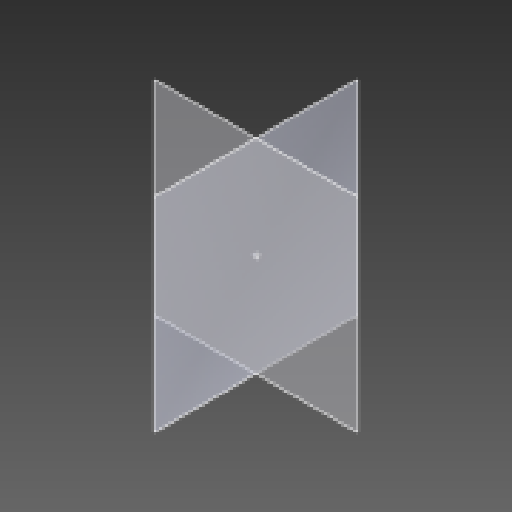
# Autodesk Inventor part: DrumstickBoundingBox
Saved by Autodesk Inventor 2023 (Build 270158000, 158)
## iProperties
Created: 2023-03-24
Part Number: DrumstickBoundingBox
Material: Generic
Document SubType Name: Modeling
Designer: Val
Density: 1 g/cm^3
Appearance: Default
Author: Val
Autodesk Inventor part; units mm, degrees
sketch "Base" plane through (0, 0, 0) normal (0, 1, 0) x (-1, 0, 0)
  arc A0 (16.4327, -16.6683) -> (16.4327, -3.9692) centre (16.3612, -10.3188) ccw projected
  circle A1 centre (16.3612, -10.3188) radius 6.35
  point P0 (0, 0)
  constraints: 1 coincident, 3 other
extrude "ForwardFeature" add sketch "Base" along normal blind 309.88 draft -0.5
sketch "Sketch2" plane through (-16.3612, 0, -10.3188) normal (0, -1, 0) x (1, 0, 0)
  circle A0 centre (0, 0) radius 6.35 projected
  point P0 (16.3612, 10.3188)
extrude "BackFeature" add sketch "Sketch2" along normal blind 88.9
sketch "Sketch3" plane through (0, 0, 0) normal (0, 1, 0) x (-1, 0, 0)
  arc A0 (16.2898, 3.9686) -> (16.4327, 3.9686) centre (16.3612, -10.3188) ccw construction
  circle A1 centre (16.3612, -10.3188) radius 14.2875
  point P0 (0, 0)
  constraints: 1 centre point, 1 coincident, 1 concentric
extrude "CollarFeature" add sketch "Sketch3" along normal mid plane 10.16
body "Solid1"
